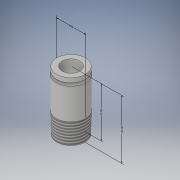
# Autodesk Inventor part: KQ2S06-01AS (A) Brass
Saved by Autodesk Inventor 2024.3 (Build 283343000, 343)
## iProperties
Created: 2023-11-03
Part Number: KQ2S06-01AS (A) Brass
Material: Generic
Catalog Web Link: www.cadenas.de
Description: KQ2S-Hex. Socket Head Male Connector (Sealant)
Vendor: SMC
Document SubType Name: Modeling
Designer: psAdmin
Manufacturer: SMC
Mass: 6.5 g
Surface Area: 11.6488 cm^2
Volume: 1.0468 cm^3
Density: 1 g/cm^3
Appearance: PSOLRGB-175-175-175
Category: PARTsolutions
Company: SMC
PSOL_IDENT_0: {$CADENAS_DATA/23d-libs/smc_jp/fittings_and_tubing/fittings_for_general_purposes/kq2_new/kq2_1/kq2s_
PSOL_IDENT_1: hshmc_s.prj},173 {VTYP=3D},{NB=KQ2S06-01AS},{LINA=KQ2S06-01AS},{NN=KQ2S},{DATE=27.10.2023 02:50:36},
PSOL_IDENT_2: {GEOMDATE=11.09.2019 04:59:54},{VERSION=},{LINEID=20},{WBVAR=MATERIAL,SEAL},{WBNUMERIC=}  {NB=KQ2S06
PSOL_IDENT_3: -01AS},{LINA=KQ2S06-01AS},{KT=DUMMY},{GUI=KQ2S06-01},{OD=6},{T=1/8},{RA=9.728},{RD=6.2},{RL=7.1},{MO
PSOL_IDENT_4: DEL=KQ2S06-01AS},{MATERIAL=A},{MATERIALX='A','(A) Brass','N','(N) Brass + With electroless nickel pl
PSOL_IDENT_5: ating'},{SEAL=S},{TUBE=06},{PORT=01},{H=4},{D=10.0},{L1=20.0},{L2=18.8},{A=16.9},{M=13.3},{EA1=10.0}
PSOL_IDENT_6: ,{EA2=9.9},{MBS=4.1},{CNSMASSEXACT=6.5},{NENN=KQ2S06-01AS},{A1=9.7},{A2=6.8},{TA=3.970},{ORDER=KQ2S0
PSOL_IDENT_7: 6-01AS}
NB: KQ2S06-01AS
NN: KQ2S
NT: Hex. Socket Head Male Connector (Sealant)
NBSYN: $MODEL.
LINA: KQ2S06-01AS
CATALOG: SMC (JP
ROWDESC: KQ2S06-01AS
GUI: KQ2S06-01
OD: 6
T: 1/8
MODEL: KQ2S06-01AS
MATERIAL: (A) Brass
SEAL: (S) With seal
H: 4
D: 10
L1: 20
L2: 18.8
A: 16.9
M: 13.3
EA1: 10
EA2: 9.9
MBS: 4.1
CNSMASSEXACT: 6.5
SUPPLIER: SMC
ARTICLENO: KQ2S06-01AS
BOMINFO: KQ2S06-01AS
CREATOR: CADENAS GmbH
Title: KQ2S06-01AS
Author: Cadenas PARTsolutions
Comments: Hex. Socket Head Male Connector (Sealant)
Autodesk Inventor part; units mm, degrees
sketch "Sketch_1" plane through (0, 0, 0) normal (0, 0, 1) x (1, 0, 0)
  line L0 (0, -3.97) -> (0, 16.9)
  line L1 (0, 16.9) -> (4.85, 16.9)
  line L2 (4.85, 16.9) -> (4.85, 15.4)
  line L3 (4.85, 15.4) -> (3.4, 15.4)
  line L4 (3.4, 15.4) -> (3.4, 14.5)
  line L5 (3.4, 14.5) -> (5, 14.5)
  line L6 (5, 14.5) -> (5, 4)
  line L7 (5, 4) -> (4.9889, 4)
  line L8 (4.9889, 4) -> (4.7401, -3.97)
  line L9 (4.7401, -3.97) -> (0, -3.97)
  line L10 (0, -3.97) -> (0, 16.9)
  constraints: 22 end point
revolve "Revolution1" add sketch "Sketch_1" angle 360 about axis through (0, -3.97, 0) along (0, -1, 0)
thread "Thread1" size "R 1/8" standard "ISO Taper" full length
sketch "_____1" plane through (0, 0, 0) normal (0, 0, 1) x (1, 0, 0)
  line L0 (-9.728, -3.1) -> (-9.728, -3.97)
  line L1 (-9.728, -3.97) -> (9.728, -3.97)
  line L2 (9.728, -3.97) -> (9.728, -3.1)
  line L3 (9.728, -3.1) -> (-9.728, -3.1)
  constraints: 8 end point
extrude "Extrusion1" cut sketch "_____1" along normal mid plane 19.456
sketch "Sketch_2" plane through (0, 0, 0) normal (0, 0, 1) x (1, 0, 0)
  line L0 (0, 3.6) -> (0, 16.9)
  line L1 (0, 16.9) -> (3, 16.9)
  line L2 (3, 16.9) -> (3, 3.6)
  line L3 (3, 3.6) -> (0, 3.6)
  line L4 (0, 3.6) -> (0, 16.9)
  constraints: 10 end point
revolve "Revolution2" cut sketch "Sketch_2" angle 360 about axis through (0, 3.6, 0) along (0, -1, 0)
sketch "Sketch_3" plane through (0, 16.9, 0) normal (0, 1, 0) x (1, 0, 0)
  line L0 (-2, -1.1547) -> (0, -2.3094)
  line L1 (0, -2.3094) -> (2, -1.1547)
  line L2 (2, -1.1547) -> (2, 1.1547)
  line L3 (2, 1.1547) -> (0, 2.3094)
  line L4 (0, 2.3094) -> (-2, 1.1547)
  line L5 (-2, 1.1547) -> (-2, -1.1547)
  constraints: 12 end point
extrude "Extrusion2" cut sketch "Sketch_3" against normal blind 18.8
ref_plane "CNS_SCREW_XY" through (0, 0, 0) normal (0, 1, 0) x (1, 0, 0)
ref_plane "CNS_SCREW_YZ" through (0, 0, 0) normal (1, 0, 0) x (0, 0, -1)
ref_plane "CNS_SCREW_ZX" through (0, 0, 0) normal (0, 0, -1) x (0, 1, 0)
body "Solid1"
